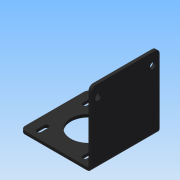
# Autodesk Inventor part: Plastina  motor
Saved by Autodesk Inventor 2017 (Build 210142000, 142)
## iProperties
Part Number: Plastina  motor
Material: Типовые
Document SubType Name: Modeling
Designer: STALKER
Density: 1 g/cm^3
Appearance: Резина — черная
Mass: 7.60598 g
Surface Area: 85.1671 cm^2
Volume: 7.60598 cm^3
Author: STALKER
Autodesk Inventor part; units mm, degrees
ref_plane "YZ Plane" through (0, 0, 0) normal (1, 0, 0) x (0, 1, 0)
ref_plane "XZ Plane" through (0, 0, 0) normal (0, 1, 0) x (-1, 0, 0)
ref_plane "XY Plane" through (0, 0, 0) normal (0, 0, 1) x (1, 0, 0)
sketch "Эскиз1" plane through (0, 0, 0) normal (0, 0, 1) x (1, 0, 0)
  circle A0 centre (0, 0) radius 12
  line L0 (0, 0) -> (0, 33) construction
  line L1 (0, 0) -> (-30.4422, 0) construction
  line L2 (-23, 23) -> (25, 23)
  line L3 (25, 23) -> (25, -23)
  line L4 (25, -23) -> (-23, -23)
  line L5 (-23, -23) -> (-23, 23)
  line L6 (15.5, 15.5) -> (-15.5, 15.5) construction
  line L7 (-15.5, 15.5) -> (-15.5, -15.5) construction
  line L8 (15.5, -15.5) -> (15.5, 15.5) construction
  line L9 (-15.5, 15.5) -> (15.5, -15.5) construction
  circle A1 centre (-15.5, 15.5) radius 1.5
  circle A2 centre (15.5, 15.5) radius 1.5
  circle A3 centre (-15.5, -15.5) radius 1.5
  circle A4 centre (15.5, -15.5) radius 1.5
  line L10 (51, 23) -> (51, -23) construction
  line L11 (-25.1704, 23) -> (21, 23) construction
  line L12 (21, -23) -> (-25.1704, -23) construction
  line L13 (-15.5, -13) -> (-15.5, -18) construction
  line L14 (-17, -13) -> (-17, -18)
  line L15 (-14, -18) -> (-14, -13)
  arc A5 (-14, -13) -> (-17, -13) centre (-15.5, -13) ccw
  arc A6 (-17, -18) -> (-14, -18) centre (-15.5, -18) ccw
  line L16 (-15.5, 18) -> (-15.5, 13) construction
  line L17 (-17, 18) -> (-17, 13)
  line L18 (-14, 13) -> (-14, 18)
  arc A7 (-14, 18) -> (-17, 18) centre (-15.5, 18) ccw
  arc A8 (-17, 13) -> (-14, 13) centre (-15.5, 13) ccw
  line L19 (15.5, 18) -> (15.5, 13) construction
  line L20 (14, 18) -> (14, 13)
  line L21 (17, 13) -> (17, 18)
  arc A9 (17, 18) -> (14, 18) centre (15.5, 18) ccw
  arc A10 (14, 13) -> (17, 13) centre (15.5, 13) ccw
  line L22 (15.5, -13) -> (15.5, -18) construction
  line L23 (14, -13) -> (14, -18)
  line L24 (17, -18) -> (17, -13)
  arc A11 (17, -13) -> (14, -13) centre (15.5, -13) ccw
  arc A12 (14, -18) -> (17, -18) centre (15.5, -18) ccw
  dimension "d0" = 24
  dimension "d1" = 31
  dimension "d2" = 31
  dimension "d3" = 3
  dimension "d4" = 3
  dimension "d5" = 3
  dimension "d6" = 3
  dimension "d7" = 46
  dimension "d51" = 48
  dimension "d52" = 23
  dimension "d53" = 8
  dimension "d54" = 8
  dimension "d55" = 8
  dimension "d56" = 8
  constraints: 58 end point, 16 point on circle, 16 tangent, 13 centre point, 8 parallel, 6 point on line, 5 coincident, 5 midpoint, 4 horizontal, 3 perpendicular, 1 collinear, 1 vertical, 1 other
  measures "d0" diameter of A0
  measures "d1" distance of L8.start L7.end
  measures "d2" distance of L7.end L6.end
  measures "d3" diameter of A1
  measures "d4" diameter of A2
  measures "d5" diameter of A3
  measures "d6" diameter of A4
  measures "d7" distance between parallel lines of L4 L2
  measures "d51" distance between parallel lines of L3 L5
  measures "d52" distance from line of L5 point (0, 0)
extrude "Выдавливание4" add sketch "Эскиз1" along normal blind 2
sketch "Эскиз3" plane through (0, 0, 2) normal (0, 0, 1) x (1, 0, 0)
  line L0 (25, -23) -> (23, -23)
  line L1 (23, -23) -> (23, 23)
  line L2 (23, 23) -> (25, 23)
  line L3 (25, 23) -> (25, -23)
  line L4 (-23, 23) -> (-23, -23) projected
  line L5 (25, -23) -> (-23, -23) projected
  line L6 (-23, 23) -> (25, 23) projected
  line L7 (25, -23) -> (25, 23) projected
  point P0 (0, 0)
  dimension "d32" = 2
  constraints: 8 end point, 3 collinear, 2 parallel, 1 horizontal, 1 perpendicular
  measures "d32" distance between parallel lines of L3 L1
extrude "Выдавливание5" add sketch "Эскиз3" along normal blind 48 contours L0 L1 L2 L3
sketch "Эскиз4" plane through (23, -23, 2) normal (-1, 0, 0) x (0, 0, 1)
  line L0 (40, 4.5) -> (40, 41.5) construction
  circle A0 centre (40, 41.5) radius 2
  circle A1 centre (40, 4.5) radius 2
  line L1 (0, 41) -> (0, 1)
  line L2 (48, 46) -> (48, 0) projected
  line L3 (48, 23) -> (59.018, 23)
  point P0 (20, 21)
  dimension "d42" = 4
  dimension "d43" = 4
  dimension "d50" = 37
  dimension "d60" = 8
  constraints: 6 end point, 2 centre point, 2 coincident, 1 horizontal, 1 midpoint, 1 symmetric about line
  measures "d42" diameter of A0
  measures "d43" diameter of A1
  measures "d50" distance of L0.end L0.start
  measures "d60" distance between parallel lines of L2 L0
extrude "Выдавливание6" cut sketch "Эскиз4" against normal blind 10
fillet "Сопряжение2" radius 1 1 edges at (23, 0, 2)
fillet "Сопряжение3" radius 3 1 edges at (25, 0, 0)
fillet "Сопряжение4" radius 3 4 edges at (-23, -23, 1) (-23, 23, 1) (24, 23, 50) (24, -23, 50)
